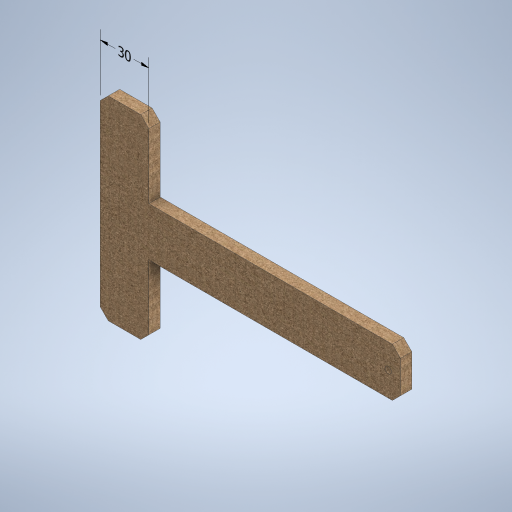
# Autodesk Inventor part: Piston
Saved by Autodesk Inventor 2023.1 (Build 271208000, 208)
## iProperties
Created: 2022-10-28
Part Number: Piston
Material: MDF Medium Density Fiberboard
Document SubType Name: Modeling
Designer: Daniel Peña
Density: 0.8 g/cm^3
Appearance: Cardboard - Corrugated
Author: Daniel Peña
Autodesk Inventor part; units mm, degrees
ref_plane "YZ Plane" through (0, 0, 0) normal (1, 0, 0) x (0, 1, 0)
ref_plane "XZ Plane" through (0, 0, 0) normal (0, 1, 0) x (-1, 0, 0)
ref_plane "XY Plane" through (0, 0, 0) normal (0, 0, 1) x (1, 0, 0)
sketch "Sketch1" plane through (0, 0, 0) normal (0, 0, 1) x (1, 0, 0)
  line L0 (100, -75) -> (100, -15) projected
  line L1 (100, 75) -> (-100, 75) projected
  line L2 (-100, 75) -> (-100, -75) projected
  line L3 (-100, -75) -> (100, -75) projected
  arc A0 (-85, -15) -> (-85, 15) centre (-85, 0) ccw projected
  line L4 (-85, 15) -> (-85, 60) projected
  line L5 (-85, 60) -> (85, 60) projected
  line L6 (85, -15) -> (85, -60) projected
  line L7 (85, -60) -> (-85, -60) projected
  line L8 (-85, -60) -> (-85, -15) projected
  line L9 (183.2183, 60) -> (203.2183, 60)
  line L10 (203.2183, -60) -> (183.2183, -60)
  line L11 (178.2183, -55) -> (178.2183, 55)
  line L12 (208.2183, 0) -> (358.2183, 0) construction
  line L13 (208.2183, 15) -> (358.2183, 15)
  line L14 (208.2183, -15) -> (358.2183, -15)
  line L15 (363.2183, -10) -> (363.2183, 10)
  line L16 (208.2183, 55) -> (208.2183, 15)
  line L17 (208.2183, -15) -> (208.2183, -55)
  line L18 (85, 60) -> (85, 15) projected
  line L19 (85, 15) -> (100, 15) projected
  line L20 (100, 15) -> (100, 75) projected
  line L21 (100, -15) -> (85, -15) projected
  line L22 (358.2183, -15) -> (363.2183, -10)
  line L23 (363.2183, 10) -> (358.2183, 15)
  line L24 (178.2183, 55) -> (183.2183, 60)
  line L25 (203.2183, 60) -> (208.2183, 55)
  line L26 (208.2183, -55) -> (203.2183, -60)
  line L27 (183.2183, -60) -> (178.2183, -55)
  point P0 (0, 0)
  point P1 (178.2183, 60)
  point P2 (208.2183, -60)
  point P3 (208.2183, 60)
  point P4 (178.2183, -60)
  point P5 (363.2183, 15)
  point P6 (363.2183, -15)
  point P7 (1.2343, 60)
  point P8 (-28.7657, -60)
  point P9 (-3.7657, -60)
  point P10 (-23.7657, -60)
  point P11 (-23.7657, 60)
  point P12 (-3.7657, 60)
  dimension "d0" = 30
  dimension "d1" = 150
  dimension "d2" = 15
  dimension "d3" = 15
  dimension "d6" = 185
  dimension "d7" = 30
  dimension "d8" = 45
  dimension "d9" = 5
  dimension "d10" = 5
  dimension "d11" = 5
  dimension "d12" = 5
  dimension "d13" = 5
  dimension "d14" = 5
  dimension "d15" = 5
  dimension "d16" = 5
  dimension "d17" = 5
  dimension "d18" = 5
  dimension "d19" = 5
  dimension "d20" = 5
  constraints: 30 end point, 14 point on line, 5 parallel, 2 horizontal, 2 perpendicular, 1 vertical
  measures "d0" distance of point (208.218, -60) point (178.218, -60)
  measures "d1" distance of L12.start L12.end
  measures "d2" distance between parallel lines of L12 L13
  measures "d3" distance between parallel lines of L12 L14
  measures "d6" distance between parallel lines of L15 L11
  measures "d7" distance between parallel lines of L11 L16
  measures "d8" distance of L14.start point (208.218, -60)
  measures "d9" distance of L14.end point (363.218, -15)
  measures "d10" distance of L15.start point (363.218, -15)
  measures "d11" distance of L15.end point (363.218, 15)
  measures "d12" distance of L13.end point (363.218, 15)
  measures "d13" distance of L11.end point (178.218, 60)
  measures "d14" distance of L9.start point (178.218, 60)
  measures "d15" distance of L9.end point (208.218, 60)
  measures "d16" distance of L16.start point (208.218, 60)
  measures "d17" distance of L17.end point (208.218, -60)
  measures "d18" distance of L10.start point (208.218, -60)
  measures "d19" distance of L10.end point (178.218, -60)
  measures "d20" distance of L11.start point (178.218, -60)
extrude "Extrusion1" add sketch "Sketch1" along normal blind 7 contours L9 L25 L16 L13 L23 L15 L22 L14 L17 L26 L10 L27 L11 L24
sketch "Sketch2" plane through (0, 0, 7) normal (0, 0, 1) x (1, 0, 0)
  line L0 (363.2183, -10) -> (363.2183, 10) projected
  point P0 (0, 0)
  point P1 (355.7183, 0)
  dimension "d21" = 7.5
  measures "d21" distance from line of L0 point (355.718, 0)
hole "Hole1" at (355.7183, 0, 7) direction (0, 0, -1) diameter 4 end through all
equation "\"d1\" = lPiston"
equation "\"d10\" = d9"
equation "\"d11\" = d9"
equation "\"d12\" = d11"
equation "\"d13\" = d9"
equation "\"d14\" = d13"
equation "\"d15\" = d9"
equation "\"d16\" = d15"
equation "\"d17\" = d9"
equation "\"d18\" = d17"
equation "\"d19\" = d9"
equation "\"d20\" = d19"
equation "\"lPiston\" = 150"
body "Solid1"
